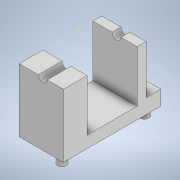
# Autodesk Inventor part: Support_1B
Saved by Autodesk Inventor 2021 (Build 250183000, 183)
## iProperties
Created: 2021-04-14
Part Number: Support_1B
Material: Generic
Document SubType Name: Modeling
Designer: Jawal
Density: 1 g/cm^3
Appearance: Default
Author: Jawal
Autodesk Inventor part; units mm, degrees
ref_plane "YZ Plane" through (0, 0, 0) normal (1, 0, 0) x (0, 1, 0)
ref_plane "XZ Plane" through (0, 0, 0) normal (0, 1, 0) x (-1, 0, 0)
ref_plane "XY Plane" through (0, 0, 0) normal (0, 0, 1) x (1, 0, 0)
sketch "Sketch1" plane through (0, 0, 0) normal (1, 0, 0) x (0, 1, 0)
  line L0 (12.0091, 20) -> (-9.4679, 20)
  line L1 (-9.4679, 20) -> (-9.4679, -13)
  line L2 (-9.4679, -13) -> (12.0091, -13)
  line L3 (12.0091, -13) -> (12.0091, 20)
  point P0 (0, 0)
  dimension "d0" = 33
  dimension "d1" = 21.477
  dimension "d14" = 20
  constraints: 8 end point, 2 parallel, 1 horizontal, 1 perpendicular
  measures "d0" distance of L0.end L1.end
  measures "d1" distance of L1.end L2.end
  measures "d14" distance from line of L0 point (0, 0)
extrude "Extrusion1" add sketch "Sketch1" along normal blind 15
sketch "Sketch2" plane through (0, -9.4679, -13) normal (0, -1, 0) x (1, 0, 0)
  circle A0 centre (12, 30.5) radius 1.5
  line L0 (0, 33) -> (15, 33) projected
  circle A1 centre (12, 2.5) radius 1.5
  line L1 (15, 33) -> (15, 0) projected
  point P0 (0, 13)
  dimension "d4" = 3
  dimension "d5" = 2.5
  dimension "d6" = 3
  dimension "d7" = 28
  dimension "d8" = 3
  dimension "d9" = 3
  constraints: 2 centre point
  measures "d4" diameter of A0
  measures "d5" distance from line of L0 A0.centre
  measures "d6" diameter of A1
  measures "d7" distance of A0.centre A1.centre
  measures "d8" distance from line of A1.centre L1
  measures "d9" distance from line of L1 A0.centre
extrude "Extrusion2" add sketch "Sketch2" along normal blind 3
sketch "Sketch3" plane through (15, 0, 0) normal (1, 0, 0) x (0, 0, -1)
  line L0 (13, 12.0091) -> (-20, 12.0091) projected
  line L1 (-12, 12.0091) -> (5, 12.0091)
  line L2 (5, 12.0091) -> (5, -5.48)
  line L3 (5, -5.48) -> (-12, -5.48)
  line L4 (-12, -5.48) -> (-12, 12.0091)
  line L5 (-20, 12.0091) -> (-20, -9.4679) projected
  line L6 (13, -9.4679) -> (13, 12.0091) projected
  point P0 (0, 0)
  point P1 (5, 12.0091)
  dimension "d12" = 8
  dimension "d13" = 8
  constraints: 8 end point, 2 parallel, 1 horizontal, 1 perpendicular, 1 point on line
  measures "d12" distance between parallel lines of L5 L4
  measures "d13" distance between parallel lines of L6 L2
extrude "Extrusion3" cut sketch "Sketch3" against normal through all
sketch "Sketch4" plane through (0, -9.4679, -13) normal (0, 0, -1) x (-1, 0, 0)
  line L0 (0, 21.477) -> (-15, 21.477) projected
  arc A0 (-9.517, 21.477) -> (-6.517, 21.477) centre (-8.017, 21.477) ccw
  line L1 (-15, 0) -> (-15, 21.477) projected
  point P0 (0, 9.4679)
  dimension "d17" = 3
  dimension "d18" = 6.983
  constraints: 3 point on line, 2 point on circle, 1 centre point
  measures "d17" diameter of A0
  measures "d18" distance from line of L1 A0.centre
extrude "Extrusion4" cut sketch "Sketch4" against normal through all
sketch "Sketch5" plane through (0, 12.0091, -5) normal (0, 1, 0) x (1, 0, 0)
  point P0 (0, -5)
sketch "Sketch6" plane through (0, -9.4679, -13) normal (0, 0, -1) x (-1, 0, 0)
  line L0 (-9.517, 21.477) -> (-15, 21.477) projected
  line L1 (-15, 21.477) -> (0, 21.477)
  line L2 (0, 21.477) -> (0, 5)
  line L3 (0, 5) -> (-15, 5)
  line L4 (-15, 5) -> (-15, 21.477)
  line L5 (0, 0) -> (-15, 0) projected
  point P0 (0, 9.4679)
  dimension "d21" = 5
  constraints: 8 end point, 2 parallel, 1 horizontal, 1 perpendicular
  measures "d21" distance between parallel lines of L5 L3
extrude "Extrusion5" cut sketch "Sketch6" against normal blind 5
equation "\"d9\" = d8"
body "Solid1"
